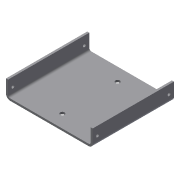
# Autodesk Inventor part: Part156
Saved by Autodesk Inventor 2014 SP2 (Build 180246200, 246)
## iProperties
Created: 2014-12-15
Part Number: Part156
Material: Generic
Document SubType Name: Sheet Metal
Designer: Admin
Density: 1 g/cm^3
Sheet Metal Rule: Default
Appearance: Default
Author: Admin
Autodesk Inventor part; units mm, degrees
ref_plane "YZ Plane" through (0, 0, 0) normal (1, 0, 0) x (0, 1, 0)
ref_plane "XZ Plane" through (0, 0, 0) normal (0, 1, 0) x (-1, 0, 0)
ref_plane "XY Plane" through (0, 0, 0) normal (0, 0, 1) x (1, 0, 0)
sketch "Sketch1" plane through (0, 0, 0) normal (0, 1, 0) x (-1, 0, 0)
  line L0 (0, 0) -> (127, 0)
  line L1 (127, 0) -> (127, 118.999)
  line L2 (127, 118.999) -> (0, 118.999)
  line L3 (0, 118.999) -> (0, 0)
  dimension "d0" = 127
  dimension "d1" = 118.999
  measures "d0" distance of L2.end L1.end
  measures "d1" distance of L1.end L0.end
extrude "Plate1" add sketch "Sketch1" along normal blind 3.048
sketch "Sketch2" plane through (-123.952, 0, 118.999) normal (-1, 0, 0) x (0, -1, 0)
  line L0 (0, -118.999) -> (0, 0)
  line L1 (0, 0) -> (-25.4, 0)
  line L2 (-25.4, 0) -> (-25.4, -118.999)
  line L3 (-25.4, -118.999) -> (0, -118.999)
  constraints: 6 end point, 1 horizontal, 1 perpendicular, 1 vertical
edge flange "Flange1" height 25.4 angle 90 thickness 3.048 bend radius 3.048 thickness toward (-1, 0, 0) relief tear relief width 3.048 relief depth 1.524 edges at (-127, 3.048, 59.4995) wall of the first edge with corners at (-123.952, 0, 0) (-123.952, 0, 118.999) (-123.952, 25.4, 118.999) (-123.952, 25.4, 0)
bend "Bend1"
corner "Corner1"
sketch "Sketch3" plane through (-3.048, 0, 0) normal (1, 0, 0) x (0, 1, 0)
  line L0 (0, 118.999) -> (0, 0)
  line L1 (0, 0) -> (25.4, 0)
  line L2 (25.4, 0) -> (25.4, 118.999)
  line L3 (25.4, 118.999) -> (0, 118.999)
  constraints: 6 end point, 1 horizontal, 1 perpendicular, 1 vertical
edge flange "Flange2" height 25.4 angle 90 thickness 3.048 bend radius 3.048 thickness toward (1, 0, 0) relief tear relief width 3.048 relief depth 1.524 edges at (0, 3.048, 59.4995) wall of the first edge with corners at (-3.048, 0, 118.999) (-3.048, 0, 0) (-3.048, 25.4, 0) (-3.048, 25.4, 118.999)
bend "Bend2"
corner "Corner2"
sketch "Sketch4" plane through (0, 3.048, 0) normal (0, 1, 0) x (1, 0, 0)
  line L0 (-120.904, 0) -> (-6.096, 0) projected
  line L1 (-6.096, -118.999) -> (-120.904, -118.999) projected
  point P0 (0, 0)
  point P1 (-63.5, -99.949)
  point P2 (-63.5, -19.05)
  dimension "d23" = 19.05
  dimension "d24" = 19.05
  measures "d23" distance from line of L0 point (-63.5, -19.05)
  measures "d24" distance from line of L1 point (-63.5, -99.949)
hole "Hole1" at (-63.5, 3.048, 99.949) at (-63.5, 3.048, 19.05) direction (0, -1, 0) diameter 6.35 end through all
sketch "Sketch5" plane through (-127, 25.4, 0) normal (-1, 0, 0) x (0, 0, 1)
  line L0 (118.999, 0) -> (118.999, -19.304) projected
  line L1 (0, -19.304) -> (0, 0) projected
  line L2 (118.999, -25.4) -> (0, -25.4) projected
  point P0 (7.112, -12.7)
  point P1 (111.887, -12.7)
  dimension "d32" = 7.112
  dimension "d33" = 7.112
  dimension "d34" = 12.7
  dimension "d35" = 12.7
  measures "d32" distance from line of point (7.112, -12.7) L1
  measures "d33" distance from line of L0 point (111.887, -12.7)
  measures "d34" distance from line of point (7.112, -12.7) L2
  measures "d35" distance from line of L2 point (111.887, -12.7)
hole "Hole2" at (-127, 12.7, 7.112) at (-127, 12.7, 111.887) direction (1, 0, 0) diameter 4.2926 depth 1016 tip angle 118
equation "\"d30\" = Thickness"
equation "\"d3\" = BendReliefWidth"
equation "\"d4\" = BendReliefDepth"
equation "\"d5\" = MinimumRemnant"
equation "\"d6\" = BendRadius"
equation "\"d9\" = BendRadius"
equation "\"d10\" = CornerReliefSize"
equation "\"d11\" = GapSize"
equation "\"d12\" = JacobiRadiusSize"
equation "\"d13\" = BendReliefWidth"
equation "\"d14\" = BendReliefDepth"
equation "\"d15\" = MinimumRemnant"
equation "\"d16\" = BendRadius"
equation "\"d19\" = BendRadius"
equation "\"d20\" = CornerReliefSize"
equation "\"d21\" = GapSize"
equation "\"d22\" = JacobiRadiusSize"
equation "\"BendRadius\" = Thickness"
equation "\"BendReliefWidth\" = Thickness"
equation "\"BendReliefDepth\" = 0.5 * Thickness"
equation "\"CornerReliefSize\" = 4 * Thickness"
equation "\"MinimumRemnant\" = 2 * Thickness"
equation "\"TransitionRadius\" = BendRadius"
equation "\"JacobiRadiusSize\" = BendRadius"
equation "\"GapSize\" = Thickness"
equation "\"d2\" = BendRadius"
equation "\"Thickness\" = 3.048"
body "Solid1"
